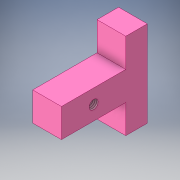
# Autodesk Inventor part: vexSupportForArm
Saved by Autodesk Inventor 2016 SP1 (Build 200210100, 210)
## iProperties
Created: 2015-07-13
Part Number: vexSupportForArm
Material: Aluminum 6061
Document SubType Name: Modeling
Designer: steele
Density: 2.7 g/cm^3
Appearance: Pink
Mass: 94.7579 g
Surface Area: 105.47 cm^2
Volume: 35.0955 cm^3
Author: steele
Autodesk Inventor part; units mm, degrees
ref_plane "YZ Plane" through (0, 0, 0) normal (1, 0, 0) x (0, 1, 0)
ref_plane "XZ Plane" through (0, 0, 0) normal (0, 1, 0) x (-1, 0, 0)
ref_plane "XY Plane" through (0, 0, 0) normal (0, 0, 1) x (1, 0, 0)
sketch "Sketch1" plane through (0, 0, 0) normal (0, 0, 1) x (1, 0, 0)
  line L0 (-6.35, -19.05) -> (6.35, -19.05)
  line L1 (6.35, -19.05) -> (6.35, 19.05)
  line L2 (6.35, 19.05) -> (-6.35, 19.05)
  line L3 (-6.35, 19.05) -> (-6.35, -19.05)
  line L4 (-6.35, -19.05) -> (6.35, 19.05) construction
  line L5 (6.35, -19.05) -> (-6.35, 19.05) construction
  point P0 (0, 0)
  dimension "height" = 38.1
  dimension "width" = 12.7
  constraints: 12 end point, 2 midpoint, 2 parallel, 1 horizontal, 1 perpendicular
  measures "height" distance of L0.end L1.end
  measures "width" distance of L1.end L2.end
extrude "Extrusion9" add sketch "Sketch1" against normal blind 9.525
sketch "Sketch19" plane through (0, 0, 0) normal (0, 0, 1) x (1, 0, 0)
  line L0 (-6.35, -6.35) -> (6.35, -6.35)
  line L1 (6.35, -6.35) -> (6.35, 6.35)
  line L2 (6.35, 6.35) -> (-6.35, 6.35)
  line L3 (-6.35, 6.35) -> (-6.35, -6.35)
  line L4 (-6.35, -6.35) -> (6.35, 6.35) construction
  line L5 (6.35, -6.35) -> (-6.35, 6.35) construction
  line L6 (-6.35, 19.05) -> (-6.35, -19.05) projected
  point P0 (0, 0)
  dimension "d126" = 12.7
  constraints: 12 end point, 2 midpoint, 2 parallel, 1 collinear, 1 perpendicular
  measures "d126" distance of L2.end L0.start
extrude "Extrusion10" add sketch "Sketch19" along normal blind 28.448
sketch "Sketch20" plane through (6.35, -19.05, -9.525) normal (1, 0, 0) x (0, 0, -1)
  line L0 (-9.525, 25.4) -> (-9.525, 38.1) projected
  line L1 (-9.525, 19.05) -> (-37.973, 19.05) construction
  line L2 (-37.973, 25.4) -> (-37.973, 12.7) construction
  point P0 (-23.749, 19.05)
  dimension "d129" = 14.224
  dimension "d137" = 0
  constraints: 2 end point, 1 midpoint
  measures "d129" distance from line of point (-23.749, 19.05) L0
  measures "d137" distance from line of point (-23.749, 19.05) L1
hole "Hole13" at (6.35, 0, 14.224) direction (-1, 0, 0) diameter 3.9624 end through all thread size "10-32 UNF" class "2B" standard "ANSI Unified Screw Threads"
equation "\"height\" = partHeight"
equation "\"width\" = partWidth"
equation "\"d124\" = depthBehindPlate"
equation "\"d126\" = slotWidth"
equation "\"d127\" = 2 * centerLineOfCylinder"
equation "\"d129\" = centerLineOfCylinder"
equation "\"partWidth\" = 12.7"
equation "\"centerLineOfCylinder\" = 14.224"
equation "\"partHeight\" = 38.1"
equation "\"depthBehindPlate\" = 9.525"
equation "\"slotWidth\" = 12.7"
body "Solid2"
